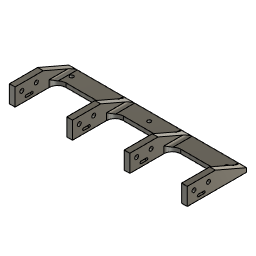
V4+Solenoid+Hanger (Autodesk Fusion 360 design; units mm, degrees)
Autodesk Fusion 360 part; units mm, degrees
note: some values were not read from the file. Set by a fixed rule: which sketch regions a step uses.
sketch "Sketch1" plane through (0, 0, 0) normal (0, 0, 1) x (1, 0, 0)
  line L0 (0, 0) -> (5, 0)
  line L1 (5, 0) -> (5, 37.75)
  line L2 (0, 52.75) -> (0, 0)
  line L3 (51, 37.75) -> (51, 0)
  line L4 (51, 0) -> (56, 0)
  line L5 (56, 0) -> (56, 37.75)
  line L6 (102, 37.75) -> (102, 0)
  line L7 (102, 0) -> (107, 0)
  line L8 (107, 0) -> (107, 37.75)
  line L9 (153, 37.75) -> (153, 0)
  line L10 (153, 0) -> (158, 0)
  line L11 (158, 0) -> (158, 52.75)
  line L12 (0, 52.75) -> (158, 52.75)
  line L13 (51, 37.75) -> (5, 37.75)
  line L14 (153, 37.75) -> (107, 37.75)
  line L15 (102, 37.75) -> (56, 37.75)
  line L16 (0, 45.25) -> (158, 45.25) construction
  circle A0 centre (10, 45.25) radius 1.625
  circle A1 centre (79, 45.25) radius 1.625
  circle A2 centre (148, 45.25) radius 1.625
  dimension "d2" = 52.75
  dimension "d10" = 7.5
  dimension "d11" = 3.25
  dimension "d12" = 10
  dimension "d13" = 10
  dimension "d25" = 15
  constraint horizontal L0
  constraint vertical L1
  constraint vertical L2
  constraint coincident L0.start L2.end
  constraint horizontal L12
  constraint horizontal L14
  constraint coincident L3.start L14
  constraint collinear L13 L14
  constraint coincident L6.start L14
  constraint collinear L14 L15
  constraint coincident L2 L16.start
  constraint coincident L11 L16.end
  constraint perpendicular L11 L16
  constraint coincident L16 A0.centre
  constraint midpoint L16 A1.centre
  constraint coincident L16 A2.centre
  constraint equal A0 A1
  constraint equal A0 A2
  measures "d2" distance of L0.start L2.start
  measures "d10" distance of L12 L16
  measures "d11" diameter of A1
  measures "d12" distance of L16.start A0.centre
  measures "d13" distance of L11 A2.centre
  measures "d25" distance of L12 L13
extrude "Extrude1" add sketch "Sketch1" along normal blind 3.5 makes body 1
sketch "Sketch2" plane through (0, 0, 0) normal (-1, 0, 0) x (0, -1, 0)
  line L0 (-52.75, 0) -> (0, 0)
  line L1 (0, 0) -> (0, 3.5)
  line L2 (0, 3.5) -> (-52.75, 3.5)
  line L3 (-52.75, 3.5) -> (-52.75, 0)
  line L4 (0, 3.5) -> (0, 15.5)
  line L5 (0, 15.5) -> (-25, 15.5)
  line L6 (0, 9.5) -> (-18.95, 9.5) construction
  circle A0 centre (-6.05, 9.5) radius 1.75
  circle A1 centre (-18.95, 9.5) radius 1.75
  line L7 (-25, 15.5) -> (-52.75, 3.5)
  dimension "d16" = 25
  dimension "d19" = 9.5
  dimension "d20" = 3.5
  dimension "d23" = 6.05
  dimension "d24" = 12.9
  dimension "d26" = 15.5
  constraint coincident L1.end L2.start
  constraint perpendicular L2 L4
  constraint perpendicular L4 L5
  constraint coincident L4 L6.start
  constraint perpendicular L4 L6
  constraint coincident L6 A0.centre
  constraint coincident L6 A1.centre
  constraint equal A0 A1
  constraint coincident L6.end A1.centre
  constraint coincident L2.end L3.start
  measures "d16" distance of L4.end L5.end
  measures "d19" distance of L0 L6
  measures "d20" diameter of A0
  measures "d23" distance of L4 A0.centre
  measures "d24" distance of A0.centre L6.end
  measures "d26" distance of L0 L5
extrude "Extrude2" add sketch "Sketch2" against normal blind 5 separate body contours L2 L4 L5 L7 makes body 2
pattern_linear "R-Pattern1" count 4 spacing 51 along (1, 0, 0) of bodies 2 makes body 3 at (51, 32.7908, 9.3281) makes body 4 at (102, 32.7908, 9.3281) makes body 5 at (153, 32.7908, 9.3281)
combine "Combine1" operation add target body 1 tool bodies 2 3 4 5
fillet "Fillet2" radius 7.5 6 edges at (5, 37.75, 1.75) (51, 37.75, 1.75) (56, 37.75, 1.75) (102, 37.75, 1.75) (107, 37.75, 1.75) (153, 37.75, 1.75) on bodies 1
fillet "Fillet3" radius 2.5 6 edges at (102, 41.5, 3.5) (51, 41.5, 3.5) (153, 41.5, 3.5) (5, 41.5, 3.5) (56, 41.5, 3.5) (107, 41.5, 3.5) on bodies 1
sketch "Sketch3" plane through (158, 0, 0) normal (1, 0, 0) x (0, 1, 0)
  circle A0 centre (6.05, 9.5) radius 1.75
  circle A1 centre (18.95, 9.5) radius 1.75
  line L0 (0, 0) -> (52.75, 0)
  line L1 (52.75, 0) -> (52.75, 3.5)
  line L2 (52.75, 3.5) -> (25, 15.5)
  line L3 (25, 15.5) -> (0, 15.5)
  line L4 (0, 15.5) -> (0, 0)
  line L5 (6.05, 9.5) -> (18.95, 9.5) construction
  line L6 (12.5, 9.5) -> (12.5, 3.5) construction
  line L7 (10, 2.5) -> (15, 2.5)
  arc A2 (15, 2.5) -> (15, 4.5) centre (15, 3.5) ccw
  line L8 (15, 4.5) -> (10, 4.5)
  arc A3 (10, 4.5) -> (10, 2.5) centre (10, 3.5) ccw
  line L9 (10, 3.5) -> (15, 3.5) construction
  point P0 (12.5, 3.5)
  dimension "d39" = 3.5
  dimension "d40" = 2.5
  dimension "d41" = 1
  constraint coincident A0.centre L5.start
  constraint coincident A1.centre L5.end
  constraint midpoint L5 L6.start
  constraint perpendicular L5 L6
  constraint tangent L7 A2
  constraint tangent A2 L8
  constraint parallel L7 L8
  constraint tangent L8 A3
  constraint tangent L7 A3
  constraint perpendicular L6 L9
  constraint coincident P0 L6.end
  constraint midpoint L9 P0
  measures "d39" distance of L0 P0
  measures "d40" distance of A2.centre P0
  measures "d41" radius of A2
extrude "Extrude3" cut sketch "Sketch3" against normal blind 160 contours L7 A2 L8 A3 bodies 1
equation "d2 = 36.25 mm + 15 mm + 1.5 mm"
equation "d23 = 4.55 mm + 1.5 mm"
